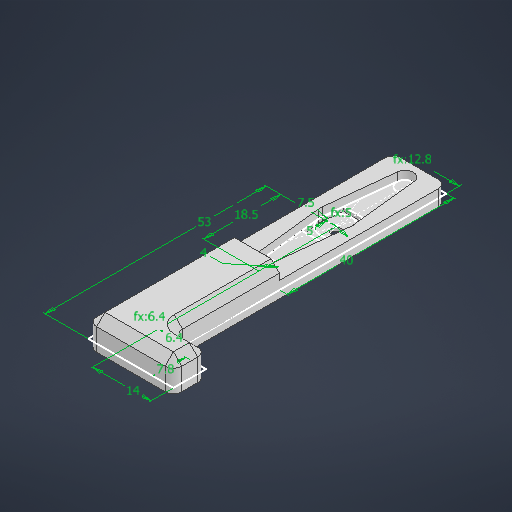
# Autodesk Inventor part: arm2
Saved by Autodesk Inventor 2025.1 (Build 291241000, 241)
## iProperties
Created: 2025-02-19
Part Number: arm2
Material: Generic
Document SubType Name: Modeling
Designer: jerem
Density: 1 g/cm^3
Appearance: Default
Author: jerem
## iProperties of the stored document arm2_3DPrint.ipt
Created: 2025-02-19
Part Number: arm2_3DPrint
Material: Generic
Document SubType Name: Modeling
Designer: jerem
Density: 1 g/cm^3
Appearance: Default
Author: jerem
Autodesk Inventor part; units mm, degrees
ref_plane "YZ Plane" through (0, 0, 0) normal (1, 0, 0) x (0, 1, 0)
ref_plane "XZ Plane" through (0, 0, 0) normal (0, 1, 0) x (-1, 0, 0)
ref_plane "XY Plane" through (0, 0, 0) normal (0, 0, 1) x (1, 0, 0)
sketch "Sketch1" plane through (0, 0, 0) normal (0, 1, 0) x (-1, 0, 0)
  circle A0 centre (0, 0) radius 3.75
  circle A1 centre (0, 16.5) radius 2
  line L0 (0, 16.5) -> (0, 0) construction
  line L1 (1.9887, 16.7121) -> (3.7288, 0.3977)
  line L2 (-3.7288, 0.3977) -> (-1.9887, 16.7121)
  line L3 (0, 16.5) -> (0, 18.5) construction
  line L4 (0, 0) -> (3.75, 0) construction
  circle A2 centre (0, -16.5) radius 2
  line L5 (0, -16.5) -> (0, -18.5) construction
  line L6 (1.9887, -16.7121) -> (3.7288, -0.3977)
  line L7 (0, -16.5) -> (0, 0) construction
  line L8 (-3.7288, -0.3977) -> (-1.9887, -16.7121)
  line L9 (3.238, 5) -> (-3.238, 5)
  line L10 (-3.238, -5) -> (3.238, -5)
  line L11 (-6.4, -20) -> (6.4, -20)
  line L12 (6.4, -20) -> (6.4, 20)
  line L13 (6.4, 20) -> (-6.4, 20)
  line L14 (-6.4, 20) -> (-6.4, -20)
  line L15 (-6.4, -20) -> (6.4, 20) construction
  line L16 (6.4, -20) -> (-6.4, 20) construction
  line L17 (6.4, 53) -> (-14, 53)
  line L18 (-14, 53) -> (-14, 45.2)
  line L19 (-14, 45.2) -> (-6.4, 45.2)
  line L20 (-6.4, 45.2) -> (-6.4, 20)
  line L21 (6.4, 53) -> (6.4, 20)
  line L22 (0, 20) -> (0, 53) construction
  point P0 (-3.7288, -0.3977)
  point P1 (3.7288, -0.3977)
  dimension "d0" = 4
  dimension "d1" = 7.5
  dimension "d2" = 18.5
  dimension "d3" = 5
  dimension "d4" = 5
  dimension "d7" = 12.8
  dimension "d8" = 40
  dimension "d9" = 6.4
  dimension "d10" = 6.4
  dimension "d11" = 53
  dimension "d12" = 14
  dimension "d13" = 7.8
  constraints: 46 end point, 9 point on circle, 9 point on line, 6 perpendicular, 6 symmetric about line, 4 horizontal, 4 tangent, 3 centre point, 3 midpoint, 3 parallel, 2 coincident, 1 vertical, 1 other
  measures "d0" diameter of A1
  measures "d1" diameter of A0
  measures "d2" distance of point (0, 0) L3.end
  measures "d3" distance from line of L9 point (0, 0)
  measures "d4" distance from line of point (0, 0) L10
  measures "d7" distance of L11.start L11.end
  measures "d8" distance of L13.end L11.start
  measures "d9" distance between parallel lines of L20 L22
  measures "d10" distance between parallel lines of L21 L22
  measures "d11" distance from line of point (0, 0) L17
  measures "d12" distance from line of L18 point (0, 0)
  measures "d13" distance between parallel lines of L17 L19
extrude "Extrusion1" add sketch "Sketch1" against normal blind 1.8 contours A0 | A0 L2 L9 L1 | L6 L10 L8 A0 | L9 L2 A1 L1 | L6 A2 L8 L10 | A1 | A2 | L14 L13 L12 L11 | L20 L19 L18 L17 L21 L13
extrude "Extrusion2" add sketch "Sketch1" along normal blind 2 contours L14 L13 L12 L11
hole "Hole2" at (0, 0, 0) direction (0, -1, 0) diameter 2.3 end through all
extrude "Extrusion3" cut sketch "Sketch1" against normal blind 1 contours A0 | A0 L2 L9 L1 | L6 L10 L8 A0
extrude "Extrusion4" add sketch "Sketch1" along normal blind 5.5 contours L20 L19 L18 L17 L21 L13
fillet "Fillet1" radius 2 6 edges at (6.4, 1.85, 45.2) (14, 1.85, 45.2) (14, 1.85, 53) (-6.4, 1.85, 53) (6.4, 0.1, -20) (-6.4, 0.1, -20)
chamfer "Chamfer1" distance 2 angle 45 8 edges at (6.4, 5.5, 31.6) (10.2, 5.5, 45.2) (13.4142, 5.5, 45.7858) (14, 5.5, 49.1) (13.4142, 5.5, 52.4142) (3.8, 5.5, 53) (-5.8142, 5.5, 52.4142) (-6.4, 5.5, 35.5)
equation "\"d4\" = d3"
equation "\"d7\" = 2 * d9"
equation "\"d10\" = d9"
body "Solid1"
